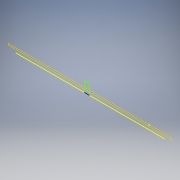
# Autodesk Inventor part: Z limit switch holder
Saved by Autodesk Inventor 2019 (Build 230136000, 136)
## iProperties
Created: 2020-08-13
Part Number: Z limit switch holder
Material: Generic
Document SubType Name: Modeling
Designer: Vijay
Density: 1 g/cm^3
Appearance: Default
Author: Vijay
Autodesk Inventor part; units mm, degrees
ref_plane "YZ Plane" through (0, 0, 0) normal (1, 0, 0) x (0, 1, 0)
ref_plane "XZ Plane" through (0, 0, 0) normal (0, 1, 0) x (-1, 0, 0)
ref_plane "XY Plane" through (0, 0, 0) normal (0, 0, 1) x (1, 0, 0)
ref_plane "Work Plane1" through (0, 0, 0) normal (0, 0, 1) x (1, 0, 0)
sketch "Sketch1" plane through (0, 0, 0) normal (0, 0, 1) x (1, 0, 0)
  line L0 (100, -28) -> (-900, -28) projected
  line L1 (-439.1083, -28) -> (-403.2461, -28)
  line L2 (-403.2461, -28) -> (-403.2461, 37.4845)
  line L3 (-403.2461, 37.4845) -> (-439.1083, 37.4845)
  line L4 (-439.1083, 37.4845) -> (-439.1083, -28)
  point P0 (0, 0)
  constraints: 8 end point, 2 parallel, 1 horizontal, 1 perpendicular, 1 point on line
extrude "Extrusion1" add sketch "Sketch1" along normal blind 4
fillet "Fillet1" radius 2 4 edges at (-439.1083, -28, 2) (-403.2461, -28, 2) (-439.1083, 37.4845, 2) (-403.2461, 37.4845, 2)
sketch "Sketch2" plane through (0, 0, 4) normal (0, 0, 1) x (1, 0, 0)
  line L0 (100, -17.1) -> (-900, -17.1) projected
  line L1 (100, -8.9) -> (100, -17.1) projected
  line L2 (100, -8.9) -> (-900, -8.9) projected
  line L3 (-900, -17.1) -> (-900, -8.9) projected
  line L4 (-900, -13) -> (100, -13) construction
  line L5 (-437.1083, -28) -> (-405.2461, -28) construction
  line L6 (-421.1772, -28) -> (-421.1772, 37.4845) construction
  line L7 (-405.2461, 37.4845) -> (-437.1083, 37.4845) construction
  circle A0 centre (-433.1083, -13) radius 3.1
  line L8 (-439.1083, 35.4845) -> (-439.1083, -26) construction
  circle A1 centre (-409.2461, -13) radius 3.1
  point P0 (0, 0)
  dimension "d3" = 6.2
  dimension "d4" = 6
  constraints: 4 end point, 4 midpoint, 2 centre point, 1 point on line, 1 symmetric about line, 1 other
  measures "d3" diameter of A0
  measures "d4" distance from line of L8 A0.centre
extrude "Extrusion2" cut sketch "Sketch2" against normal through all contours A0 | A1
sketch "Sketch3" plane through (0, 0, 4) normal (0, 0, 1) x (1, 0, 0)
  line L0 (-438.583, 11.7754) -> (-438.5811, 14.7754) projected
  arc A0 (-438.583, 11.7754) -> (-436.5842, 9.7741) centre (-436.583, 11.7741) ccw projected
  line L1 (-433.5842, 9.7722) -> (-436.5842, 9.7741) projected
  line L2 (-433.5823, 12.7722) -> (-433.5842, 9.7722) projected
  arc A1 (-433.5823, 12.7722) -> (-435.5811, 14.7735) centre (-435.5823, 12.7735) ccw projected
  line L3 (-438.5811, 14.7754) -> (-435.5811, 14.7735) projected
  line L4 (-437.6826, 12.2748) -> (-437.6822, 13.0248) projected
  arc A2 (-434.4822, 13.0228) -> (-437.6822, 13.0248) centre (-436.0822, 13.0238) ccw projected
  line L5 (-434.4822, 13.0228) -> (-434.4827, 12.2728) projected
  arc A3 (-437.6826, 12.2748) -> (-434.4827, 12.2728) centre (-436.0827, 12.2738) ccw projected
  line L6 (-423.4684, 34.7658) -> (-423.4703, 31.7658) projected
  arc A4 (-423.4684, 34.7658) -> (-425.4671, 36.7671) centre (-425.4684, 34.7671) ccw projected
  line L7 (-428.4671, 36.769) -> (-425.4671, 36.7671) projected
  line L8 (-428.469, 33.769) -> (-428.4671, 36.769) projected
  arc A5 (-428.469, 33.769) -> (-426.4703, 31.7677) centre (-426.469, 33.7677) ccw projected
  line L9 (-423.4703, 31.7658) -> (-426.4703, 31.7677) projected
  circle A6 centre (-425.9687, 34.2674) radius 1.6 projected
  point P0 (0, 0)
extrude "Extrusion3" cut sketch "Sketch3" against normal through all contours L4 A2 L5 A3 | A6
sketch "Sketch4" plane through (0, 0, 4) normal (0, 0, 1) x (1, 0, 0)
  line L0 (-394.0939, 43.6118) -> (-422.77, 43.6118)
  line L1 (-422.77, 43.6118) -> (-422.77, 2.3518)
  line L2 (-422.77, 2.3518) -> (-394.0939, 2.3518)
  line L3 (-394.0939, 2.3518) -> (-394.0939, 43.6118)
  point P0 (0, 0)
  constraints: 8 end point, 2 parallel, 1 horizontal, 1 perpendicular
extrude "Extrusion4" cut sketch "Sketch4" against normal through all
fillet "Fillet2" radius 2 3 edges at (-403.2461, 2.3518, 2) (-422.77, 37.4845, 2) (-422.77, 2.3518, 2)
body "Solid1"
